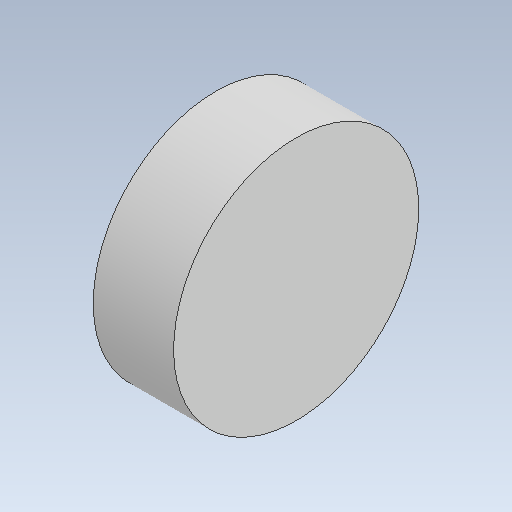
# Autodesk Inventor part: WHEEL
Saved by Autodesk Inventor 2020 (Build 240168000, 168)
## iProperties
Created: 2021-01-07
Part Number: WHEEL
Material: Generic
Document SubType Name: Modeling
Designer: lucky
Density: 1 g/cm^3
Appearance: Default
Mass: 912.073 g
Surface Area: 604.219 cm^2
Volume: 912.073 cm^3
Author: lucky
Autodesk Inventor part; units mm, degrees
ref_plane "YZ Plane" through (0, 0, 0) normal (1, 0, 0) x (0, 1, 0)
ref_plane "XZ Plane" through (0, 0, 0) normal (0, 1, 0) x (-1, 0, 0)
ref_plane "XY Plane" through (0, 0, 0) normal (0, 0, 1) x (1, 0, 0)
sketch "Sketch1" plane through (0, 0, 0) normal (1, 0, 0) x (0, 1, 0)
  circle A0 centre (0, 0) radius 76.2
  dimension "d0" = 152.4
  constraints: 1 centre point, 1 coincident
  measures "d0" diameter of A0
extrude "Extrusion1" add sketch "Sketch1" along normal blind 50
equation "\"d0\" = Wheel_Diametre"
equation "\"Chassi_CentreDrop\" = 4"
equation "\"WheelBay_Depth\" = 55"
equation "\"Chassi_GroundClearance\" = 10.116"
equation "\"Wheel_Diametre\" = 152.4"
equation "\"Wheel_Seperation\" = 285.75"
equation "\"Wheel_HeightOffset\" = 4"
equation "\"Wheel_Clearance\" = 13.05"
equation "\"Wheel_CentreDrop\" = 4"
equation "\"Wheel_Seperation2\" = 194.33333"
equation "\"Wheel_HeightOffset2\" = 4"
equation "\"Wheel_Diametre2\" = 101.6"
equation "\"Wheel_Clearance2\" = 32.7"
equation "\"Chain_Pitch\" = 9.525"
equation "\"Wheel_MaxSeperation\" = 285.75"
equation "\"Wheel_CCSpan\" = 571.5"
equation "\"Wheel_CCSpan2\" = 471.5"
equation "\"Wheel_MaxSeperation2\" = 190.5"
equation "\"MotorholeHorizontal\" = 95.01318"
equation "\"Chassi_SideRivetSpacing\" = 37.5"
equation "\"OutputshaftTopOffset\" = 30.058"
equation "\"MotorholeCC\" = 95.25"
equation "\"Heightfromcenter\" = 6.7125"
equation "\"Sprocket_Thickness\" = 10.668"
equation "\"BumperMountingBarOffset\" = 177.8"
body "Solid1"
